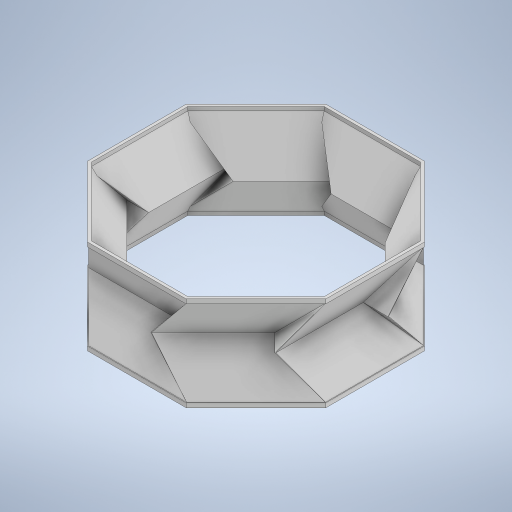
# Autodesk Inventor part: 팔각형 OV-PAM 층 한개
Saved by Autodesk Inventor 2024 (Build 280153000, 153)
## iProperties
Created: 2023-06-16
Part Number: 팔각형 OV-PAM 층 한개
Material: 일반
Document SubType Name: Modeling
Designer: jsw
Density: 1 g/cm^3
Appearance: 기본값
Author: jsw
Autodesk Inventor part; units mm, degrees
ref_plane "YZ Plane" through (0, 0, 0) normal (1, 0, 0) x (0, 1, 0)
ref_plane "XZ Plane" through (0, 0, 0) normal (0, 1, 0) x (-1, 0, 0)
ref_plane "XY Plane" through (0, 0, 0) normal (0, 0, 1) x (1, 0, 0)
sketch "스케치1" plane through (0, 0, 0) normal (0, 1, 0) x (-1, 0, 0)
  line L0 (-32.591883, 13.5) -> (-13.5, 32.591883)
  line L1 (-13.5, 32.591883) -> (13.5, 32.591883)
  line L2 (13.5, 32.591883) -> (32.591883, 13.5)
  line L3 (32.591883, 13.5) -> (32.591883, -13.5)
  line L4 (32.591883, -13.5) -> (13.5, -32.591883)
  line L5 (13.5, -32.591883) -> (-13.5, -32.591883)
  line L6 (-13.5, -32.591883) -> (-32.591883, -13.5)
  line L7 (-32.591883, -13.5) -> (-32.591883, 13.5)
  line L8 (-13.748528, 33.191883) -> (13.748528, 33.191883)
  line L9 (13.748528, 33.191883) -> (33.191883, 13.748528)
  line L10 (33.191883, 13.748528) -> (33.191883, -13.748528)
  line L11 (33.191883, -13.748528) -> (13.748528, -33.191883)
  line L12 (13.748528, -33.191883) -> (-13.748528, -33.191883)
  line L13 (-13.748528, -33.191883) -> (-33.191883, -13.748528)
  line L14 (-33.191883, -13.748528) -> (-33.191883, 13.748528)
  line L15 (-33.191883, 13.748528) -> (-13.748528, 33.191883)
  point P0 (0, 0)
  point P1 (0, 0)
  point P2 (0, 0)
  dimension "d0" = 27
  dimension "d2" = 0.6
  constraints: 32 end point, 2 coincident, 2 horizontal, 34 other
  measures "d0" distance of L0.end L1.end
  measures "d2" distance between parallel lines of L10 L3
extrude "돌출2" add sketch "스케치1" along normal blind 12 contours L0 L1 L2 L3 L4 L5 L6 L7 | L8 L9 L10 L11 L12 L13 L14 L15
ref_plane "작업 평면2" through (33.191883, 0, 13.748528) normal (-0.8660254, -0.5, 0) x (0, 0, -1)
sketch "스케치3" plane through (33.191883, 0, 13.748528) normal (1, 0, 0) x (0, 0, -1)
  line L0 (0, 0) -> (0, 12)
  line L1 (0, 12) -> (27.497056, 12)
  line L2 (0, 0) -> (27.497056, 0)
  line L3 (27.497056, 0) -> (27.497056, 12)
  line L4 (27.497056, 12) -> (0, 12)
  line L5 (0, 12) -> (0, 0)
  line L6 (0, 12) -> (-7.304723, 12)
  line L7 (-19.443355, 12) -> (0, 12)
  line L8 (0, 0) -> (-7.304723, 12)
  line L9 (27.497056, 12) -> (13.748528, 12)
  line L10 (17.497056, 12) -> (27.497056, 0)
  point P0 (13.748528, 0)
  point P1 (17.497056, 12)
  dimension "d17" = 121.33
  dimension "d53" = 10
  constraints: 16 end point, 5 midpoint, 2 parallel, 2 point on line, 1 horizontal, 1 perpendicular
  measures "d17" angle of L8 L2
  measures "d53" distance of L10.start L1.end
extrude "돌출4" cut sketch "스케치3" against normal up to surface contours L8 L6 L0 | L0 L1 L10 L2 surface through (33.191883, 0, 13.748528) normal (-0.8660254, -0.5, 0)
pattern_circular "원형 패턴1" count 8 over 360 about axis through (0, -10, 0) along (0, 1, 0) of "돌출4"
mirror "미러5" about plane through (0, 12, 0) normal (0, 1, 0) of "돌출2", "돌출4", "원형 패턴1"
sketch "스케치9" plane through (-13.748528, 24, -33.191883) normal (0, 1, 0) x (1, 0, 0)
  line L0 (46.940411, -46.940411) -> (46.940411, -19.443355)
  line L1 (46.940411, -19.443355) -> (27.497056, 0)
  line L2 (27.497056, 0) -> (0, 0)
  line L3 (0, 0) -> (-19.443355, -19.443355)
  line L4 (-19.443355, -19.443355) -> (-19.443355, -46.940411)
  line L5 (-19.443355, -46.940411) -> (0, -66.383766)
  line L6 (0, -66.383766) -> (27.497056, -66.383766)
  line L7 (27.497056, -66.383766) -> (46.940411, -46.940411)
  point P0 (13.748528, -33.191883)
extrude "돌출8" add sketch "스케치9" along normal blind 1.2
sketch "스케치10" plane through (0, 0, 0) normal (0, -1, 0) x (1, 0, 0)
  line L0 (33.191883, 13.748528) -> (33.191883, -13.748528)
  line L1 (13.748528, 33.191883) -> (33.191883, 13.748528)
  line L2 (-13.748528, 33.191883) -> (13.748528, 33.191883)
  line L3 (-33.191883, 13.748528) -> (-13.748528, 33.191883)
  line L4 (-33.191883, -13.748528) -> (-33.191883, 13.748528)
  line L5 (-13.748528, -33.191883) -> (-33.191883, -13.748528)
  line L6 (13.748528, -33.191883) -> (-13.748528, -33.191883)
  line L7 (33.191883, -13.748528) -> (13.748528, -33.191883)
  point P0 (0, 0)
extrude "돌출9" add sketch "스케치10" along normal blind 1.2
shell "쉘6" thickness 0.6 removed faces 2 at (4.582843, 25.2, 11.063961) at (4.582843, -1.2, -1.898276)
sketch "스케치12" plane through (-13.748528, 25.2, -33.191883) normal (0, 1, 0) x (1, 0, 0)
  line L0 (46.340411, -19.691883) -> (46.340411, -46.691883)
  line L1 (46.340411, -46.691883) -> (27.248528, -65.783766)
  line L2 (27.248528, -65.783766) -> (0.248528, -65.783766)
  line L3 (0.248528, -65.783766) -> (-18.843355, -46.691883)
  line L4 (-18.843355, -46.691883) -> (-18.843355, -19.691883)
  line L5 (-18.843355, -19.691883) -> (0.248528, -0.6)
  line L6 (0.248528, -0.6) -> (27.248528, -0.6)
  line L7 (27.248528, -0.6) -> (46.340411, -19.691883)
  line L8 (46.940411, -19.443355) -> (27.497056, 0)
  line L9 (27.497056, 0) -> (0, 0)
  line L10 (0, 0) -> (-19.443355, -19.443355)
  line L11 (-19.443355, -19.443355) -> (-19.443355, -46.940411)
  line L12 (-19.443355, -46.940411) -> (0, -66.383766)
  line L13 (0, -66.383766) -> (27.497056, -66.383766)
  line L14 (27.497056, -66.383766) -> (46.940411, -46.940411)
  line L15 (46.940411, -46.940411) -> (46.940411, -19.443355)
  line L16 (-0.082843, 0.2) -> (27.579899, 0.2)
  line L17 (27.579899, 0.2) -> (47.140411, -19.360512)
  line L18 (47.140411, -19.360512) -> (47.140411, -47.023254)
  line L19 (47.140411, -47.023254) -> (27.579899, -66.583766)
  line L20 (27.579899, -66.583766) -> (-0.082843, -66.583766)
  line L21 (-0.082843, -66.583766) -> (-19.643355, -47.023254)
  line L22 (-19.643355, -47.023254) -> (-19.643355, -19.360512)
  line L23 (-19.643355, -19.360512) -> (-0.082843, 0.2)
  point P0 (13.748528, -33.191883)
  point P1 (13.748528, -33.191883)
  dimension "d50" = 0.2
  constraints: 16 end point, 1 coincident, 1 horizontal, 17 other
  measures "d50" distance between parallel lines of L9 L16
extrude "돌출10" add sketch "스케치12" against normal blind 1.2 contours L16 L17 L18 L19 L20 L21 L22 L23
ref_plane "작업 평면6" through (-13.748528, 12, -33.191883) normal (0, 1, 0) x (1, 0, 0)
mirror "미러8" about plane through (-13.748528, 12, -33.191883) normal (0, 1, 0) of "돌출10"
